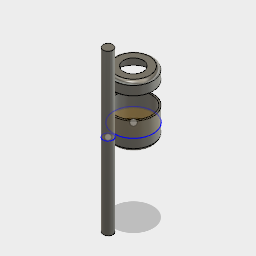
JPHACKS v3 (Autodesk Fusion 360 design; units mm, degrees)
Autodesk Fusion 360 part; units mm, degrees
form "フォーム1" [no effect]
sketch "スケッチ1" plane through (0, 0, 0) normal (0, 1, 0) x (1, 0, 0)
  circle A0 centre (0, 0) radius 15.2697
extrude "押し出し1" add sketch "スケッチ1" along normal blind 239.614 makes body 1
move_face "面をオフセット1" offset 252.9308 1 faces at (2.4345, 0, 9.1829) on bodies 1
sketch "スケッチ2" plane through (0, 0, 0) normal (0, 1, 0) x (1, 0, 0)
  circle A0 centre (0, 78.425) radius 60.1784
extrude "押し出し2" add sketch "スケッチ2" against normal blind 37.4056 separate body makes body 2
fillet "フィレット1" radius 9.84 1 edges at (-56.106, -37.4056, -100.1864) on bodies 2
copy_body "ボディのコピーと貼り付け1" bodies 2 makes body 3
move_body "ボディを移動1" bodies 3 to x (1, 0, 0) y (0, 1, 0) z (0, 0, 1) at (0, 123.8306, 0)
move_body "ボディを移動2" bodies 3 to x (-1, 0, 0) y (0, -1, 0) z (0, 0, 1) at (-0.3784, 236.9631, 0)
shell "シェル2" thickness 5 removed faces 1 at (-4.8421, 113.1324, -58.8684) on bodies 3
hole "穴1" at (-0.3784, 113.1324, -78.425) direction (0, 1, 0) diameter 73.931 depth 33.232 tip angle 118 bodies 3
move_face "面をオフセット2" offset 46.137 1 faces at (4.4637, 0, -58.8684) on bodies 2
shell "シェル1" thickness 5 removed faces 1 at (4.4637, 46.137, -58.8684) on bodies 2
